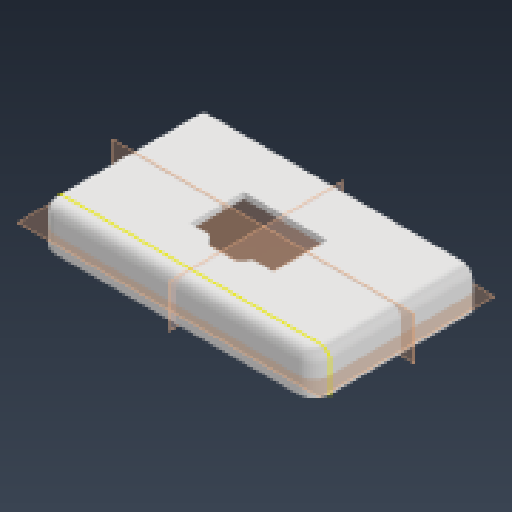
# Autodesk Inventor part: Крышка_электроники
Saved by Autodesk Inventor 2023.2 (Build 272271030, 271C)
## iProperties
Created: 2025-12-29
Part Number: Крышка_электроники
Material: Типовые
Document SubType Name: Modeling
Designer: Олег Коноваленко
Density: 1 g/cm^3
Appearance: По умолчанию
Author: Олег Коноваленко
Autodesk Inventor part; units mm, degrees
sketch "Эскиз1" plane through (0, 0, 0) normal (0, 0, 1) x (1, 0, 0)
  line L0 (-70, -15) -> (-70, 18)
  line L1 (-70, 18) -> (70, 18)
  line L2 (70, 18) -> (70, -15)
  line L3 (70, -15) -> (67, -15)
  line L4 (67, -15) -> (67, 15)
  line L5 (67, 15) -> (-67, 15)
  line L6 (-67, 15) -> (-67, -15)
  line L7 (-67, -15) -> (-70, -15)
  line L8 (0, 24.6) -> (0, -21.6) construction
  line L9 (-98, 0) -> (98, 0) projected
  circle A0 centre (62, 10) radius 5
  circle A1 centre (65, 13) radius 5
  circle A2 centre (-65, 13) radius 5
  circle A3 centre (-62, 10) radius 5
  point P0 (0, 0)
  point P1 (0, 18)
  point P2 (-67, 0)
  point P3 (62, 15)
  point P4 (67, 10)
  point P5 (70, 13)
  point P6 (65, 18)
  point P7 (-67, 10)
  point P8 (-62, 15)
  point P9 (-65, 18)
  point P10 (-70, 13)
  dimension "d0" = 134
  dimension "d2" = 3
  dimension "d3" = 3
  dimension "d4" = 33
  dimension "d8" = 10
  constraints: 16 end point, 8 tangent, 6 perpendicular, 4 centre point, 3 equal radius, 2 equal length, 2 midpoint, 2 point on line, 1 parallel, 1 vertical
  measures "d0" distance between parallel lines of L4 L6
  measures "d2" distance between parallel lines of L5 L1
  measures "d3" distance between parallel lines of L2 L4
  measures "d4" distance of L0.start L0.end
  measures "d8" diameter of A0
extrude "Выдавливание1" add sketch "Эскиз1" along normal mid plane 72.75 contours L0 L9 L6 L7 | L0 A2 L6 L9 | A2 L5 L6 | L1 A1 L5 A2 | L9 L2 L3 L4 | L4 A1 L2 L9 | A1 L4 L5 | L6 L5 A3 | A0 L5 L4
sketch "Эскиз3" plane through (0, 0, 36.375) normal (0, 0, 1) x (1, 0, 0)
  arc A0 (67, 10) -> (62, 15) centre (62, 10) ccw projected
  line L0 (62, 15) -> (62, 18)
  line L1 (65, 18) -> (-65, 18) projected
  arc A1 (70, 13) -> (65, 18) centre (65, 13) ccw projected
  line L2 (70, -15) -> (70, 13) projected
  line L3 (67, -15) -> (70, -15) projected
  line L4 (67, 10) -> (67, -15) projected
  arc A2 (-62, 15) -> (-67, 10) centre (-62, 10) ccw projected
  line L5 (-67, -15) -> (-67, 10) projected
  line L6 (-70, -15) -> (-67, -15) projected
  line L7 (-70, 13) -> (-70, -15) projected
  arc A3 (-65, 18) -> (-70, 13) centre (-65, 13) ccw projected
  line L8 (-62, 15) -> (62, 15) projected
  line L9 (-62, 15) -> (-62, 18)
  point P0 (0, 0)
  constraints: 4 end point, 2 point on line, 2 vertical
revolve "Вращение1" add sketch "Эскиз3" angle 90 about axis through (-62, 15, 36.375) along (0, 1, 0) contours A2 L5 L6 L7 A3 L1 L9
revolve "Вращение2" add sketch "Эскиз3" angle 90 about axis through (62, 15, 36.375) along (0, -1, 0) contours A0 L0 L1 A1 L2 L3 L4
sketch "Эскиз4" plane through (62, 15, 36.375) normal (-1, 0, 0) x (0, 0, 1)
  line L0 (3, 3) -> (0, 3) projected
  line L1 (0, 0) -> (0, 3) projected
  arc A0 (5, -5) -> (0, 0) centre (0, -5) ccw projected
  line L2 (5, -5) -> (5, -30) projected
  line L3 (5, -30) -> (8, -30) projected
  line L4 (8, -30) -> (8, -2) projected
  arc A1 (8, -2) -> (3, 3) centre (3, -2) ccw projected
  point P0 (-36.375, -15)
extrude "Выдавливание2" add sketch "Эскиз4" along normal up to surface (124 mm away)
sketch "Эскиз5" plane through (-65, 18, -36.375) normal (0, 1, 0) x (1, 0, 0)
  line L0 (43.75, -52.75) -> (86.25, -52.75)
  line L1 (86.25, -52.75) -> (86.25, -25.35)
  line L2 (86.25, -25.35) -> (43.75, -25.35)
  line L3 (43.75, -25.35) -> (43.75, -52.75)
  line L4 (43.75, -52.75) -> (86.25, -25.35) construction
  line L5 (86.25, -52.75) -> (43.75, -25.35) construction
  line L6 (65, 14.55) -> (65, -87.3) construction
  line L7 (59.875, -52.75) -> (70.125, -52.75) construction
  line L8 (59.875, -47.75) -> (70.125, -47.75)
  line L9 (70.125, -57.75) -> (59.875, -57.75)
  arc A0 (59.875, -47.75) -> (59.875, -57.75) centre (59.875, -52.75) ccw
  arc A1 (70.125, -57.75) -> (70.125, -47.75) centre (70.125, -52.75) ccw
  line L10 (3, -72.75) -> (127, -72.75) projected
  circle A2 centre (46.025, -22.55) radius 1.4
  circle A3 centre (83.975, -22.55) radius 1.4
  circle A4 centre (46.025, -55.55) radius 1.4
  circle A5 centre (83.975, -55.55) radius 1.4
  line L11 (46.025, -22.55) -> (46.025, -55.55) construction
  line L12 (46.025, -55.55) -> (83.975, -55.55) construction
  line L13 (83.975, -55.55) -> (83.975, -22.55) construction
  line L14 (83.975, -22.55) -> (46.025, -22.55) construction
  line L15 (46.025, -22.55) -> (83.975, -55.55) construction
  line L16 (83.975, -22.55) -> (46.025, -55.55) construction
  point P0 (65, -36.375)
  point P1 (65, -52.75)
  point P2 (75.125, -52.75)
  point P3 (54.875, -52.75)
  point P4 (54.875, -52.75)
  point P5 (75.125, -52.75)
  point P6 (65, -39.05)
  dimension "d13" = 27.4
  dimension "d14" = 42.5
  dimension "d15" = 5
  dimension "d16" = 20.25
  dimension "d17" = 15
  dimension "d21" = 2.8
  dimension "d22" = 37.95
  dimension "d23" = 33
  constraints: 32 end point, 6 centre point, 6 point on circle, 5 midpoint, 4 perpendicular, 4 tangent, 3 equal radius, 3 parallel, 3 point on line, 1 horizontal, 1 vertical
  measures "d13" distance of L0.end L1.end
  measures "d14" distance of L1.end L2.end
  measures "d15" distance between parallel lines of L9 L0
  measures "d16" distance of point (75.125, -52.75) point (54.875, -52.75)
  measures "d17" distance between parallel lines of L10 L9
  measures "d21" diameter of A2
  measures "d22" distance of L13.end L11.start
  measures "d23" distance of L12.end L13.end
extrude "Выдавливание3" cut sketch "Эскиз5" against normal up to next
fillet "Сопряжение2" radius 2 2 edges at (-10.125, 16.5, 16.375) (10.125, 16.5, 16.375)
sketch "Эскиз6" plane through (-70, -15, -36.375) normal (0, -1, 0) x (1, 0, 0)
  line L0 (147.5, 7.5) -> (147.5, 20.5) construction
  line L1 (155, 7.5) -> (155, 20.5)
  line L2 (140, 20.5) -> (140, 7.5)
  arc A0 (140, 7.5) -> (155, 7.5) centre (147.5, 7.5) ccw
  arc A1 (155, 20.5) -> (140, 20.5) centre (147.5, 20.5) ccw
  line L3 (140, 0) -> (140, 72.75) projected
  line L4 (147.5, 0) -> (140, 0)
  line L5 (140, 0) -> (140, 72.75) projected
  line L6 (147.5, 28) -> (140, 28)
  circle A2 centre (147.5, 7.5) radius 1.5
  circle A3 centre (147.5, 20.5) radius 1.5
  circle A4 centre (150, 37.8205) radius 10
  point P0 (70, 36.375)
  point P1 (147.5, 14)
  point P2 (140, 15)
  point P3 (140, 7.5)
  point P4 (148.5714, 27.9231)
  point P5 (140, 37.8205)
  dimension "d24" = 13
  dimension "d25" = 7.5
  dimension "d27" = 3
  dimension "d32" = 20
  constraints: 12 end point, 6 point on circle, 6 tangent, 5 centre point, 4 point on line, 2 coincident, 2 perpendicular, 1 equal radius, 1 midpoint, 1 parallel, 1 vertical
  measures "d24" distance of L0.start L0.end
  measures "d25" distance between parallel lines of L1 L0
  measures "d27" diameter of A2
  measures "d32" diameter of A4
extrude "Выдавливание4" add sketch "Эскиз6" against normal blind 7 contours A0 L2 A1 L1 | L4 L3 A0 | A1 L6 L3 A4 | A1 L3 L6
mirror "Зеркальное отражение1" about plane through (0, 0, 0) normal (1, 0, 0) of "Выдавливание4"
fillet "Сопряжение4" radius 1 2 edges at (-70, -8, -17.4647) (70, -8, -17.4647)
